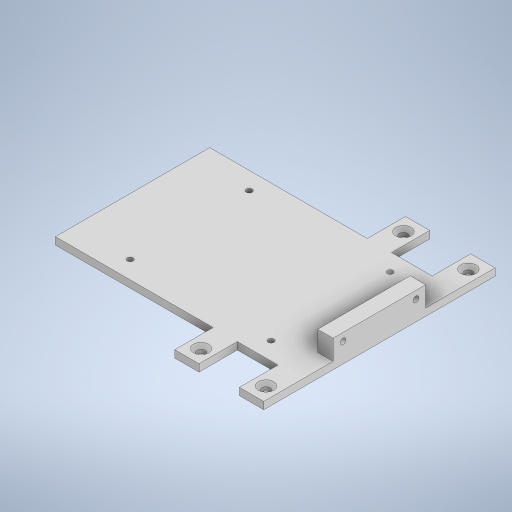
# Autodesk Inventor part: OT2-ridingcam-r1
Saved by Autodesk Inventor 2024.1 (Build 281209000, 209)
## iProperties
Created: 2024-06-04
Part Number: OT2-ridingcam-r1
Material: Generic
Document SubType Name: Modeling
Designer: pab2
Density: 1 g/cm^3
Appearance: Default
Author: pab2
Autodesk Inventor part; units mm, degrees
ref_plane "YZ Plane" through (0, 0, 0) normal (1, 0, 0) x (0, 1, 0)
ref_plane "XZ Plane" through (0, 0, 0) normal (0, 1, 0) x (-1, 0, 0)
ref_plane "XY Plane" through (0, 0, 0) normal (0, 0, 1) x (1, 0, 0)
sketch "Sketch1" plane through (0, 0, 0) normal (0, 1, 0) x (-1, 0, 0)
  line L0 (-5, 47.5) -> (5, 47.5)
  line L1 (5, 47.5) -> (5, -47.5)
  line L2 (5, -47.5) -> (-5, -47.5)
  line L3 (-5, -47.5) -> (-5, 47.5)
  line L4 (-5, 47.5) -> (5, -47.5) construction
  line L5 (5, 47.5) -> (-5, -47.5) construction
  line L6 (-31.75, 31.75) -> (31.75, 31.75)
  line L7 (31.75, 31.75) -> (31.75, -31.75)
  line L8 (31.75, -31.75) -> (-31.75, -31.75)
  line L9 (-31.75, -31.75) -> (-31.75, 31.75)
  line L10 (-31.75, 31.75) -> (31.75, -31.75) construction
  line L11 (31.75, 31.75) -> (-31.75, -31.75) construction
  line L12 (31.75, 31.75) -> (69.85, 31.75)
  line L13 (69.85, 31.75) -> (69.85, -31.75)
  line L14 (69.85, -31.75) -> (31.75, -31.75)
  line L15 (31.75, -31.75) -> (31.75, 31.75)
  line L16 (-31.75, 0) -> (-26.7462, 0)
  line L17 (-21.7424, 47.6123) -> (-31.75, 47.6123)
  line L18 (-31.75, 47.6123) -> (-31.75, -47.6123)
  line L19 (-31.75, -47.6123) -> (-21.7424, -47.6123)
  line L20 (-21.7424, -47.6123) -> (-21.7424, 47.6123)
  line L21 (-21.7424, 47.6123) -> (-31.75, -47.6123) construction
  line L22 (-31.75, 47.6123) -> (-21.7424, -47.6123) construction
  point P0 (0, 0)
  point P1 (-5, -31.75)
  point P2 (-5, 31.75)
  point P3 (31.75, 31.75)
  point P4 (5, 31.75)
  point P5 (5, -31.75)
  point P6 (-21.7424, -31.75)
  point P7 (-21.7424, 31.75)
  dimension "d0" = 10
  dimension "d1" = 95
  dimension "d13" = 63.5
  dimension "d14" = 63.5
  dimension "d15" = 38.1
  dimension "d47" = 5.0038
  dimension "d48" = 95.2246
  constraints: 46 end point, 8 parallel, 7 midpoint, 5 horizontal, 4 perpendicular
  measures "d0" distance of L1.end L2.end
  measures "d1" distance of L0.end L1.end
  measures "d13" distance of L7.end L8.end
  measures "d14" distance of L6.end L7.end
  measures "d15" distance of L13.end L14.end
  measures "d47" distance of L16.start L16.end
  measures "d48" distance of L18.end L17.end
extrude "Extrusion1" add sketch "Sketch1" along normal blind 3
sketch "Sketch2" plane through (0, 3, 0) normal (0, 1, 0) x (1, 0, 0)
  line L0 (0, 0) -> (0, 41.65)
  line L1 (0, 0) -> (0, -41.65)
  line L2 (21.7424, -47.6123) -> (31.75, -47.6123) projected
  line L3 (26.7462, -47.6123) -> (26.7462, 0)
  line L4 (26.7462, 0) -> (26.7462, 41.656)
  line L5 (26.7462, 0) -> (26.7462, -41.656)
  dimension "d4" = 41.65
  dimension "d5" = 41.65
  dimension "d49" = 41.656
  dimension "d50" = 41.656
  constraints: 10 end point, 3 vertical, 2 point on line, 1 midpoint
  measures "d4" distance of L0.start L0.end
  measures "d5" distance of L0.start L1.end
  measures "d49" distance of L3.end L4.end
  measures "d50" distance of L3.end L5.end
hole "Hole1" at (0, 3, 41.65) at (0, 3, -41.65) at (26.7462, 3, 41.656) at (26.7462, 3, -41.656) direction (0, -1, 0) diameter 3.4036 end through all countersink diameter 6.2992 countersink angle 90 clearance for "Flat Head Machine Screw" size "M3" standard "Ansi Metric M Profile"
sketch "Sketch3" plane through (0, 3, 0) normal (0, 1, 0) x (1, 0, 0)
  line L0 (31.75, -31.75) -> (31.75, 31.75) projected
  line L1 (31.75, 0) -> (28.575, 0)
  line L2 (25.4, -19.05) -> (31.75, -19.05)
  line L3 (31.75, -19.05) -> (31.75, 19.05)
  line L4 (31.75, 19.05) -> (25.4, 19.05)
  line L5 (25.4, 19.05) -> (25.4, -19.05)
  line L6 (25.4, -19.05) -> (31.75, 19.05) construction
  line L7 (31.75, -19.05) -> (25.4, 19.05) construction
  point P0 (0, 0)
  dimension "d16" = 3.175
  dimension "d17" = 38.1
  constraints: 14 end point, 3 midpoint, 2 horizontal, 2 parallel, 1 perpendicular, 1 point on line
  measures "d16" distance of L1.start L1.end
  measures "d17" distance of L3.end L2.end
extrude "Extrusion2" add sketch "Sketch3" along normal blind 8.255
sketch "Sketch4" plane through (31.75, 0, 31.75) normal (1, 0, 0) x (0, 0, -1)
  line L0 (12.7, 11.255) -> (50.8, 11.255) projected
  line L1 (31.75, 11.255) -> (31.75, 8.08)
  line L2 (31.75, 8.08) -> (46.75, 8.08)
  line L3 (46.75, 8.08) -> (16.75, 8.08)
  point P0 (31.75, 0)
  dimension "d20" = 3.175
  dimension "d21" = 15
  dimension "d22" = 30
  constraints: 6 end point, 1 horizontal, 1 midpoint, 1 point on line, 1 vertical
  measures "d20" distance of L1.start L1.end
  measures "d21" distance of L1.end L2.end
  measures "d22" distance of L2.end L3.end
hole "Hole2" at (31.75, 8.08, 15) at (31.75, 8.08, -15) direction (-1, 0, 0) diameter 2.3876 end through all clearance for "Flat Head Machine Screw" size "M2" standard "Ansi Metric M Profile"
sketch "Sketch5" plane through (0, 3, 0) normal (0, 1, 0) x (1, 0, 0)
  line L0 (-69.85, 31.75) -> (-69.85, -31.75) projected
  line L1 (-69.85, 0) -> (-69.85, 24.5)
  line L2 (-69.85, 24.5) -> (-69.85, -24.5)
  line L3 (-69.85, -24.5) -> (15.15, -24.5)
  line L4 (15.15, -24.5) -> (-69.85, -24.5)
  line L5 (-69.85, -24.5) -> (-69.85, 24.5)
  line L6 (-69.85, 24.5) -> (15.15, 24.5)
  line L7 (15.15, 24.5) -> (15.15, -24.5)
  line L8 (15.15, -24.5) -> (11.65, -24.5)
  line L9 (11.65, -24.5) -> (11.65, -21)
  line L10 (11.65, -21) -> (15.15, -21)
  line L11 (15.15, -21) -> (15.15, -24.5)
  line L12 (15.15, 24.5) -> (11.65, 24.5)
  line L13 (11.65, 24.5) -> (11.65, 21)
  line L14 (11.65, 21) -> (15.15, 21)
  line L15 (15.15, 21) -> (15.15, 24.5)
  line L16 (11.65, -21) -> (-46.35, -21)
  line L17 (11.65, -21) -> (69.65, -21) construction
  line L18 (11.65, 21) -> (-46.35, 21)
  line L19 (-46.35, 21) -> (-46.35, 24.5)
  line L20 (-46.35, -21) -> (-46.35, -24.5)
  point P0 (0, 0)
  dimension "d30" = 24.5
  dimension "d31" = 49
  dimension "d32" = 85
  dimension "d33" = 3.5
  dimension "d34" = 3.5
  dimension "d35" = 3.5
  dimension "d36" = 3.5
  dimension "d37" = 58
  dimension "d38" = 180
  dimension "d39" = 58
  constraints: 40 end point, 6 horizontal, 6 parallel, 5 point on line, 4 perpendicular, 1 collinear, 1 midpoint, 1 vertical
  measures "d30" distance of L1.start L1.end
  measures "d31" distance of L1.end L2.end
  measures "d32" distance of L2.end L3.end
  measures "d33" distance of L9.end L10.end
  measures "d34" distance of L8.end L9.end
  measures "d35" distance of L14.end L13.end
  measures "d36" distance of L13.end L12.end
  measures "d37" distance of L9.end L16.end
  measures "d38" angle of L16 L17
  measures "d39" distance of L13.end L18.end
hole "Hole3" at (11.65, 3, 24.5) at (11.65, 3, -24.5) at (-46.35, 3, -24.5) at (-46.35, 3, 24.5) direction (0, -1, 0) diameter 2.3876 end through all clearance for "Flat Head Machine Screw" size "M2" standard "Ansi Metric M Profile"
body "Solid1"
